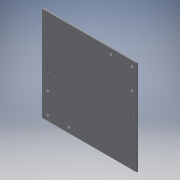
# Autodesk Inventor part: battery plate
Saved by Autodesk Inventor 2016 (Build 200138000, 138)
## iProperties
Created: 2016-02-26
Part Number: battery plate
Material: Aluminum 6061
Document SubType Name: Modeling
Designer: gus
Density: 2.7 g/cm^3
Appearance: Aluminum - Flat
Author: gus
Autodesk Inventor part; units mm, degrees
ref_plane "YZ Plane" through (0, 0, 0) normal (1, 0, 0) x (0, 1, 0)
ref_plane "XZ Plane" through (0, 0, 0) normal (0, 1, 0) x (-1, 0, 0)
ref_plane "XY Plane" through (0, 0, 0) normal (0, 0, 1) x (1, 0, 0)
sketch "Sketch1" plane through (0, 0, 0) normal (0, 0, 1) x (1, 0, 0)
  line L0 (0, 0) -> (228.6, 0)
  line L1 (228.6, 0) -> (228.6, 217.932)
  line L2 (228.6, 217.932) -> (0, 217.932)
  line L3 (0, 217.932) -> (0, 0)
  circle A0 centre (12.7, 12.7) radius 3.3734
  circle A1 centre (63.5, 12.7) radius 3.3734
  circle A2 centre (12.7, 63.5) radius 3.3734
  circle A3 centre (215.9, 154.432) radius 3.3734
  circle A4 centre (165.1, 205.232) radius 3.3734
  circle A5 centre (215.9, 205.232) radius 3.3734
  line L4 (0, 12.7) -> (228.6, 12.7) construction
  line L5 (12.7, 217.932) -> (12.7, 0) construction
  line L6 (228.6, 205.232) -> (0, 205.232) construction
  line L7 (215.9, 217.932) -> (215.9, 0) construction
  line L8 (12.7, 122.682) -> (15.875, 122.682)
  line L9 (15.875, 122.682) -> (15.875, 97.282)
  line L10 (15.875, 97.282) -> (12.7, 97.282)
  line L11 (12.7, 97.282) -> (12.7, 122.682)
  line L12 (215.9, 97.282) -> (212.725, 97.282)
  line L13 (212.725, 97.282) -> (212.725, 122.682)
  line L14 (212.725, 122.682) -> (215.9, 122.682)
  line L15 (215.9, 122.682) -> (215.9, 97.282)
  dimension "d0" = 228.6
  dimension "d1" = 217.932
  dimension "d2" = 6.7469
  dimension "d3" = 12.7
  dimension "d4" = 12.7
  dimension "d5" = 12.7
  dimension "d6" = 12.7
  dimension "d9" = 50.8
  dimension "d10" = 50.8
  dimension "d11" = 50.8
  dimension "d12" = 50.8
  dimension "d15" = 95.25
  dimension "d16" = 25.4
  dimension "d17" = 3.175
  dimension "d18" = 95.25
  constraints: 32 end point, 18 point on line, 7 perpendicular, 6 centre point, 6 parallel, 5 equal radius, 3 horizontal, 2 equal length
  measures "d0" distance of L2.end L1.end
  measures "d1" distance of L1.end L0.end
  measures "d2" diameter of A0
  measures "d3" distance between parallel lines of L2 L6
  measures "d4" distance between parallel lines of L1 L7
  measures "d5" distance between parallel lines of L0 L4
  measures "d6" distance between parallel lines of L3 L5
  measures "d9" distance of A5.centre A4.centre
  measures "d10" distance of A5.centre A3.centre
  measures "d11" distance of A0.centre A1.centre
  measures "d12" distance of A2.centre A0.centre
  measures "d15" distance between parallel lines of L2 L8
  measures "d16" distance of L8.end L9.end
  measures "d17" distance of L9.end L10.end
  measures "d18" distance between parallel lines of L2 L14
extrude "Extrusion2" add sketch "Sketch1" along normal blind 3.175
body "Solid2"
